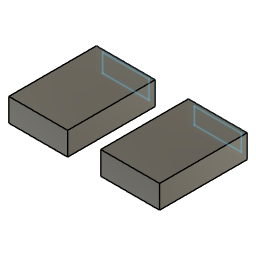
Remotes wall mounts (Autodesk Fusion 360 design; units mm, degrees)
Autodesk Fusion 360 part; units mm, degrees
sketch "Sketch1" plane through (0, 0, 0) normal (0, 0, 1) x (1, 0, 0)
  line L0 (23.5, -35) -> (-23.5, -35)
  line L1 (-23.5, -35) -> (-23.5, 35)
  line L2 (-23.5, 35) -> (23.5, 35)
  line L3 (23.5, 35) -> (23.5, -35)
  line L4 (23.5, -35) -> (-23.5, 35) construction
  line L5 (-23.5, -35) -> (23.5, 35) construction
  dimension "d1" = 70
  dimension "d2" = 47
  constraint horizontal L0
  constraint perpendicular L0 L1
  constraint parallel L0 L2
  constraint parallel L1 L3
  constraint coincident L4 origin
  constraint coincident L5 origin
  measures "d1" distance of L0 L2
  measures "d2" distance of L1 L3
extrude "Extrude1" add sketch "Sketch1" along normal blind 18.5 makes body 1
sketch "Sketch2" plane through (0, 35, 0) normal (0, 1, 0) x (-1, 0, 0)
  line L0 (-23.5, 0) -> (23.5, 0)
  line L1 (23.5, 0) -> (23.5, 18.5)
  line L2 (23.5, 18.5) -> (-23.5, 18.5)
  line L3 (-23.5, 18.5) -> (-23.5, 0)
  line L4 (18.6888, 2.8525) -> (-18.8112, 2.8525)
  line L5 (-18.8112, 2.8525) -> (-18.8112, 15.8525)
  line L6 (-18.8112, 15.8525) -> (18.6888, 15.8525)
  line L7 (18.6888, 15.8525) -> (18.6888, 2.8525)
  dimension "d5" = 13
  dimension "d6" = 37.5
  constraint horizontal L4
  constraint vertical L5
  constraint horizontal L6
  constraint vertical L7
  measures "d5" distance of L4 L6
  measures "d6" distance of L5 L7
extrude "Extrude2" cut sketch "Sketch2" against normal blind 65 contours L4 L5 L6 L7 bodies 1
sketch "Sketch3" plane through (0, 0, 18.5) normal (0, 0, 1) x (-1, 0, 0)
  line L0 (-23.5, -35) -> (23.5, -35)
  line L1 (23.5, -35) -> (23.5, 35)
  line L2 (23.5, 35) -> (-23.5, 35)
  line L3 (-23.5, 35) -> (-23.5, -35)
  line L4 (97, -35) -> (50, -35)
  line L5 (50, -35) -> (50, 35)
  line L6 (50, 35) -> (97, 35)
  line L7 (97, 35) -> (97, -35)
  dimension "d9" = 47
  dimension "d10" = 70
  constraint horizontal L4
  constraint vertical L5
  constraint horizontal L6
  constraint vertical L7
  measures "d9" distance of L5 L7
  measures "d10" distance of L4 L6
extrude "Extrude3" add sketch "Sketch3" against normal blind 18.5 separate body contours L4 L5 L6 L7 makes body 2
sketch "Sketch5" plane through (0, 35, 0) normal (0, 1, 0) x (-1, 0, 0)
  line L0 (97, 18.5) -> (50, 18.5)
  line L1 (50, 18.5) -> (50, 0)
  line L2 (50, 0) -> (97, 0)
  line L3 (97, 0) -> (97, 18.5)
  line L4 (54.9552, 16.4924) -> (91.9552, 16.4924)
  line L5 (91.9552, 16.4924) -> (91.9552, 1.9924)
  line L6 (91.9552, 1.9924) -> (54.9552, 1.9924)
  line L7 (54.9552, 1.9924) -> (54.9552, 16.4924)
  dimension "d13" = 37
  dimension "d14" = 14.5
  constraint horizontal L4
  constraint vertical L5
  constraint horizontal L6
  constraint vertical L7
  measures "d13" distance of L5 L7
  measures "d14" distance of L4 L6
extrude "Extrude4" cut sketch "Sketch5" against normal blind 65 contours L4 L5 L6 L7 bodies 2
